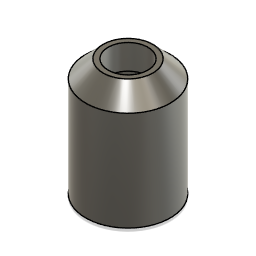
_Cap.6a81387d-0d19-46f6-b313-7a321f0e394d (Autodesk Fusion 360 design; units mm, degrees)
Autodesk Fusion 360 part; units mm, degrees
sketch "Sketch1" plane through (0, 0, 0) normal (0, 1, 0) x (1, 0, 0)
  circle A0 centre (0, 0) radius 7
  circle A1 centre (0, 0) radius 8.5
  dimension "d8" = 14
  dimension "d9" = 17
  constraint coincident A0.centre A1.centre
  constraint concentric A0 A1
  measures "d8" diameter of A0
  measures "d9" diameter of A1
extrude "Extrude1" add sketch "Sketch1" along normal blind 20 makes body 1
sketch "Sketch2" plane through (0, 20, 0) normal (0, 1, 0) x (-1, 0, 0)
  circle A0 centre (0, 0) radius 7
  circle A1 centre (0, 0) radius 8.5
sketch "Sketch3" plane through (0, 0, 0) normal (0, 0, 1) x (1, 0, 0)
  line L0 (0, 20) -> (0, 22.5)
  line L1 (-7, 20) -> (-8.5, 20)
  line L2 (-8.5, 20) -> (-5, 23.5)
  line L3 (0, 23.5) -> (0, 22.5)
  line L4 (-5, 23.5) -> (0, 23.5)
  line L5 (-7, 20) -> (0, 20)
  constraint vertical L0
  constraint perpendicular L3 L4
  constraint perpendicular L0 L5
revolve "Revolve1" add sketch "Sketch3" angle 360 about axis through (0, 1.75, 0) along (0, 1, 0) bodies 1
sketch "Sketch5" plane through (0, 23.5, 0) normal (0, 1, 0) x (-1, 0, 0)
  circle A0 centre (0, 0) radius 5
  circle A1 centre (0, 0) radius 4
  constraint concentric A0 A1
extrude "Extrude3" cut sketch "Sketch5" against normal blind 14 contours A1 bodies 1
move_body "Move1" bodies 1 to x (1, 0, 0) y (0, 1, 0) z (0, 0, 1) at (0, -5, 0)
split "Split1" by plane through (0, 0, 0) normal (0, 1, 0) bodies 1 makes body 2 at (-8.4894, 10, 0.4237)
thread "Thread3" "ISO Metric profile 14.0 M14x2 6H" major diameter 14.2505 minor diameter 12.0225 pitch 2 angle 60 modelled right hand crest width 0.5471 on face at (6.9652, -1.6667, -0.697) crest through (6.0113, -4.5, 0) on bodies 1
combine "Combine1" operation add target body 2 tool bodies 1
sketch "Sketch6" plane through (0, 0, 0) normal (0, 1, 0) x (1, 0, 0)
  circle A0 centre (0, 0) radius 7.13
  constraint coincident A0.centre origin
extrude "Extrude4" cut sketch "Sketch6" along normal blind 10 bodies 2
extrude "Extrude5" add 1 faces at (5.959, 15, 0.5465) along direction (0, -1, 0) blind 1.5 on bodies 2 bodies 2
